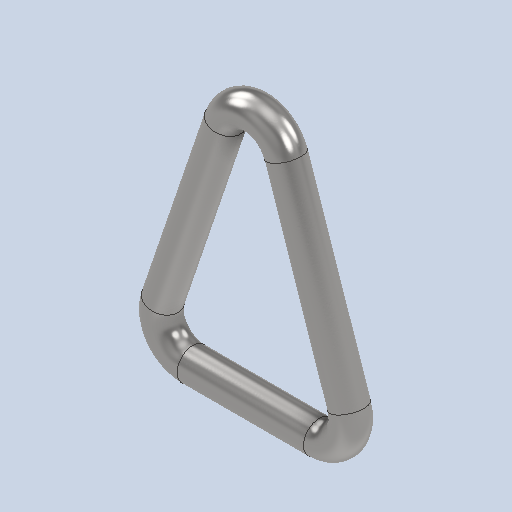
# Autodesk Inventor part: triange carabiner
Saved by Autodesk Inventor 2024 (Build 280153000, 153)
## iProperties
Created: 2023-05-23
Part Number: triange carabiner
Material: Steel, Galvanized
Document SubType Name: Modeling
Designer: Patrick
Density: 7.85 g/cm^3
Appearance: Galvanized
Author: Patrick
Autodesk Inventor part; units mm, degrees
ref_plane "YZ Plane" through (0, 0, 0) normal (1, 0, 0) x (0, 1, 0)
ref_plane "XZ Plane" through (0, 0, 0) normal (0, 1, 0) x (-1, 0, 0)
ref_plane "XY Plane" through (0, 0, 0) normal (0, 0, 1) x (1, 0, 0)
sketch "Sketch1" plane through (0, 0, 0) normal (0, 0, 1) x (1, 0, 0)
  arc A0 (9.4707, 3.2104) -> (-9.4707, 3.2104) centre (0, 0) ccw
  line L0 (9.4707, 3.2104) -> (29.4707, -55.7896)
  arc A1 (20, -69) -> (29.4707, -55.7896) centre (20, -59) ccw
  line L1 (20, -69) -> (-20, -69)
  arc A2 (-29.4707, -55.7896) -> (-20, -69) centre (-20, -59) ccw
  line L2 (-29.4707, -55.7896) -> (-9.4707, 3.2104)
  line L3 (0, 26.2863) -> (0, -87.718) projected
  point P0 (0, 10)
  dimension "d0" = 79
  dimension "d1" = 60
  dimension "d3" = 10
  constraints: 7 point on circle, 6 end point, 6 tangent, 3 centre point, 1 coincident, 1 equal radius, 1 horizontal, 1 point on line, 1 symmetric about line
  measures "d0" distance from line of point (0, 10) L1
  measures "d3" radius of A0
sketch "Sketch2" plane through (0, 0, 0) normal (1, 0, 0) x (0, 1, 0)
  circle A0 centre (10, 0) radius 5
  point P0 (0, 0)
  dimension "d4" = 10
  constraints: 1 centre point, 1 coincident
  measures "d4" diameter of A0
sweep "Sweep1" add profiles "Sketch2" path "Sketch1" path curves A0 L2 A2 L1 A1 L0
body "Solid1"
